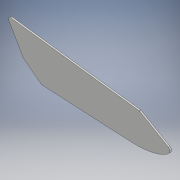
# Autodesk Inventor part: bracket
Saved by Autodesk Inventor 2018.2 (Build 222227000, 227)
## iProperties
Created: 2018-03-06
Part Number: bracket
Material: 一般
Document SubType Name: Modeling
Designer: ku_sk
Density: 1 g/cm^3
Appearance: 既定
Author: ku_sk
Autodesk Inventor part; units mm, degrees
ref_plane "YZ Plane" through (0, 0, 0) normal (1, 0, 0) x (0, 1, 0)
ref_plane "XZ Plane" through (0, 0, 0) normal (0, 1, 0) x (-1, 0, 0)
ref_plane "XY Plane" through (0, 0, 0) normal (0, 0, 1) x (1, 0, 0)
sketch "スケッチ1" plane through (0, 0, 0) normal (0, 1, 0) x (-1, 0, 0)
  line L0 (291.6076, 44.0321) -> (352.6658, 36.9174) projected
  line L1 (352.6658, 36.9174) -> (355.0856, 76.6007) projected
  line L2 (355.0856, 76.6007) -> (269.0016, 63.509) projected
  line L3 (269.0016, 63.509) -> (291.6076, 44.0321) projected
  line L4 (132.7161, 3.5142) -> (150.4021, 50.7481) projected
  line L5 (150.4021, 50.7481) -> (98.7306, 43.6255) projected
  line L6 (98.7306, 43.6255) -> (132.7161, 3.5142) projected
  line L7 (71.5255, -13.8781) -> (118.3577, -14.9798) projected
  line L8 (118.3577, -14.9798) -> (86.7096, 23.5699) projected
  line L9 (86.7096, 23.5699) -> (71.5255, -13.8781) projected
  line L10 (313.7076, -5.8004) -> (291.4126, 29.994) projected
  line L11 (291.4126, 29.994) -> (271.7097, -9.6068) projected
  line L12 (271.7097, -9.6068) -> (313.7076, -5.8004) projected
  line L13 (260.4868, 47.8263) -> (262.3081, -10.4835) projected
  line L14 (262.3081, -10.4835) -> (282.0681, 29.2322) projected
  line L15 (282.0681, 29.2322) -> (260.4868, 47.8263) projected
  line L16 (323.2812, 5.7482) -> (352.0763, 27.2481) projected
  line L17 (352.0763, 27.2481) -> (304.6777, 32.7712) projected
  line L18 (304.6777, 32.7712) -> (323.2812, 5.7482) projected
  line L19 (26.7058, 4.295) -> (56.4892, -13.5243) projected
  line L20 (56.4892, -13.5243) -> (69.1982, 26.078) projected
  line L21 (69.1982, 26.078) -> (26.7058, 4.295) projected
  line L22 (364.6383, 23.9082) -> (399.8979, 82.3649) projected
  line L23 (399.8979, 82.3649) -> (367.9521, 78.2557) projected
  line L24 (367.9521, 78.2557) -> (364.6383, 23.9082) projected
  line L25 (157.5665, 48.0655) -> (141.5591, -14.8781) projected
  line L26 (141.5591, -14.8781) -> (173.5739, -13.8781) projected
  line L27 (173.5739, -13.8781) -> (157.5665, 48.0655) projected
  line L28 (200.374, -13.041) -> (251.4069, -11.4469) projected
  line L29 (251.4069, -11.4469) -> (249.6696, 44.1742) projected
  line L30 (249.6696, 44.1742) -> (200.374, -13.041) projected
  line L31 (165.4814, 52.2118) -> (186.2732, -9.6068) projected
  line L32 (186.2732, -9.6068) -> (246.2929, 60.0555) projected
  line L33 (246.2929, 60.0555) -> (165.4814, 52.2118) projected
  circle A0 centre (322.4385, -2.626) radius 4 projected
  circle A1 centre (77.5679, 36.3106) radius 4 projected
  circle A2 centre (257.5679, 59.1248) radius 4 projected
  arc A3 (374.0171, 18.2349) -> (375.2976, 19.7024) centre (370.9621, 22.1931) ccw projected
  line L34 (329.1362, -16.4048) -> (374.0171, 18.2349) projected
  arc A4 (326.3465, -17.4396) -> (329.1362, -16.4048) centre (326.0812, -12.4466) ccw projected
  line L35 (100.5026, -29.4375) -> (326.3465, -17.4396) projected
  arc A5 (74.9408, -30.0377) -> (100.5026, -29.4375) centre (77.5861, 401.9345) ccw projected
  arc A6 (28.1912, -23.4013) -> (74.9408, -30.0377) centre (76.0159, 145.5175) ccw projected
  arc A7 (1.2395, -11.312) -> (28.1912, -23.4013) centre (55.8939, 74.446) ccw projected
  arc A8 (-6.0217, -4.7376) -> (1.2395, -11.312) centre (16.9451, 13.3315) ccw projected
  arc A9 (-3.831, 6.6355) -> (-6.0217, -4.7376) centre (0, 0) ccw projected
  line L36 (71.8122, 50.3081) -> (-3.831, 6.6355) projected
  arc A10 (73.6835, 50.9383) -> (71.8122, 50.3081) centre (74.3122, 45.978) ccw projected
  line L37 (408.3679, 93.358) -> (73.6835, 50.9383) projected
  arc A11 (413.332, 85.907) -> (408.3679, 93.358) centre (408.9966, 88.3977) ccw projected
  line L38 (413.332, 85.907) -> (375.2976, 19.7024) projected
  circle A12 centre (130.4331, -10.1322) radius 5 projected
  circle A13 centre (20.0666, -1.5588) radius 5 projected
  circle A14 centre (359.7933, 56.2153) radius 3 projected
  circle A15 centre (287.1934, 37.1564) radius 3 projected
  point P0 (0, 0)
extrude "押し出し1" add sketch "スケッチ1" along normal mid plane 4 contours L3 L2 L1 L0 | L6 L5 L4 | L9 L8 L7 | L12 L11 L10 | L15 L14 L13 | L18 L17 L16 | L21 L20 L19 | L24 L23 L22 | L27 L26 L25 | L30 L29 L28 | L33 L32 L31 | A0 | A1 | A2 | L34 A4 L35 A5 A6 A7 A8 A9 L36 A10 L37 A11 L38 A3 | A12 | A13 | A14 | A15
